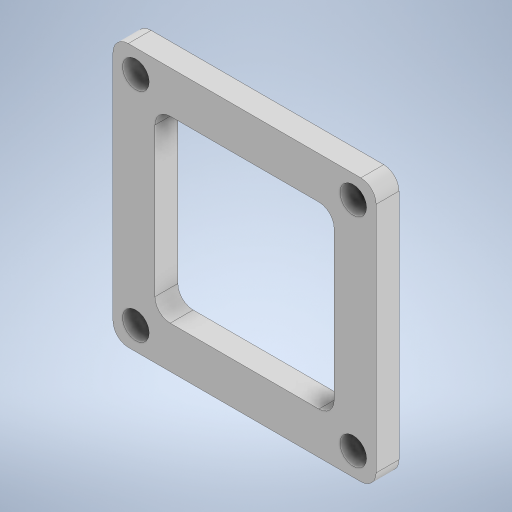
# Autodesk Inventor part: load_cell_frame
Saved by Autodesk Inventor 2024 (Build 280153000, 153)
## iProperties
Created: 2023-09-05
Part Number: load_cell_frame
Material: Generic
Document SubType Name: Modeling
Designer: Pintu
Density: 1 g/cm^3
Appearance: Default
Author: Pintu
Autodesk Inventor part; units mm, degrees
ref_plane "YZ Plane" through (0, 0, 0) normal (1, 0, 0) x (0, 1, 0)
ref_plane "XZ Plane" through (0, 0, 0) normal (0, 1, 0) x (-1, 0, 0)
ref_plane "XY Plane" through (0, 0, 0) normal (0, 0, 1) x (1, 0, 0)
sketch "Sketch1" plane through (0, 0, 0) normal (0, 0, 1) x (1, 0, 0)
  line L0 (-17.25, -17.25) -> (17.25, -17.25)
  line L1 (17.25, -17.25) -> (17.25, 17.25)
  line L2 (17.25, 17.25) -> (-17.25, 17.25)
  line L3 (-17.25, 17.25) -> (-17.25, -17.25)
  line L4 (-17.25, -17.25) -> (17.25, 17.25) construction
  line L5 (17.25, -17.25) -> (-17.25, 17.25) construction
  line L6 (11.75, -11.75) -> (-11.75, -11.75)
  line L7 (-11.75, -11.75) -> (-11.75, 11.75)
  line L8 (-11.75, 11.75) -> (11.75, 11.75)
  line L9 (11.75, 11.75) -> (11.75, -11.75)
  circle A0 centre (-14.25, -14.25) radius 1.75
  line L10 (0, -17.25) -> (0, 17.25) construction
  line L11 (-17.25, 0) -> (17.25, 0) construction
  circle A1 centre (14.25, -14.25) radius 1.75
  circle A2 centre (14.25, -14.25) radius 1.75
  circle A3 centre (-14.25, -14.25) radius 1.75
  circle A4 centre (14.25, 14.25) radius 1.75
  circle A5 centre (-14.25, 14.25) radius 1.75
  point P0 (0, 0)
  dimension "d14" = 34.5
  dimension "d15" = 34.5
  dimension "d16" = 5.5
  dimension "d17" = 3.5
  dimension "d18" = 3
  dimension "d19" = 3
  constraints: 24 end point, 6 centre point, 6 midpoint, 6 symmetric about line, 4 parallel, 2 perpendicular, 1 horizontal, 8 other
  measures "d14" distance of L2.end L1.end
  measures "d15" distance of L1.end L0.end
  measures "d16" distance between parallel lines of L0 L6
  measures "d17" diameter of A0
  measures "d18" distance from line of L0 A0.centre
  measures "d19" distance from line of L3 A0.centre
extrude "Extrusion2" add sketch "Sketch1" along normal blind 3
fillet "Fillet2" radius 2 8 edges at (-17.25, -17.25, 1.5) (-11.75, -11.75, 1.5) (-11.75, 11.75, 1.5) (-17.25, 17.25, 1.5) (17.25, 17.25, 1.5) (11.75, 11.75, 1.5) (11.75, -11.75, 1.5) (17.25, -17.25, 1.5)
body "Solid2"
